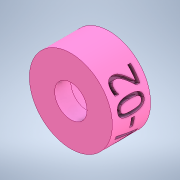
# Autodesk Inventor part: brakeLockSpacer
Saved by Autodesk Inventor 2021.1 (Build 251245000, 245)
## iProperties
Created: 2020-08-18
Part Number: brakeLockSpacer
Material: Polycarbonate, Smoke
Document SubType Name: Modeling
Designer: robst
Density: 1.2 g/cm^3
Appearance: Pink
Author: robst
Autodesk Inventor part; units mm, degrees
ref_plane "XZ Plane" through (0, 0, 0) normal (0, 1, 0) x (-1, 0, 0)
ref_plane "XY Plane" through (0, 0, 0) normal (0, 0, 1) x (1, 0, 0)
sketch "Sketch1" plane through (0, 0, 0) normal (0, 0, 1) x (1, 0, 0)
  circle A0 centre (0, 0) radius 8.0645
  circle A1 centre (0, 0) radius 20.6375
  dimension "d0" = 16.129
  dimension "d1" = 41.275
  constraints: 2 centre point, 2 coincident
  measures "d0" diameter of A0
  measures "d1" diameter of A1
extrude "Extrusion1" add sketch "Sketch1" against normal blind 19.05
sketch "Sketch3" plane through (0, 0, 0) normal (1, 0, 0) x (0, 1, 0)
  line L0 (0, 0) -> (0, -127) construction
  line L1 (-8.0645, -19.05) -> (-8.0645, 0) construction
  line L2 (-20.6375, -19.05) -> (20.6375, -19.05) construction
  line L3 (8.0645, -19.05) -> (8.0645, 0) construction
  line L4 (8.0645, -19.05) -> (8.0645, -8.0515)
  line L5 (8.0645, -8.0515) -> (14.4145, -19.05)
  line L6 (8.0645, -19.05) -> (22.7292, -19.05)
  dimension "d8" = 30
  dimension "d10" = 6.35
  constraints: 8 end point, 1 parallel, 1 point on line, 2 other
  measures "d8" angle of L5 L3
  measures "d10" distance of L5.end L3.start
revolve "Revolution1" cut sketch "Sketch3" angle 360 about axis through (0, 0, 0) along (0, 0, -1)
ref_plane "Work Plane1" through (20.6375, 0, 0) normal (1, 0, 0) x (0, 1, 0)
sketch "Sketch9" plane through (20.6375, 0, 0) normal (1, 0, 0) x (0, 1, 0)
  line L0 (20.6375, 0) -> (20.6375, -19.05) construction
  line L1 (20.6375, -9.525) -> (-20.6375, -9.525) construction
  line L2 (-20.6375, 0) -> (-20.6375, -19.05) construction
  line L3 (-7.4152, -3.175) -> (-11.7892, -15.875)
  line L4 (-11.7892, -15.875) -> (-13.6108, -15.875)
  line L5 (-13.6108, -15.875) -> (-17.9848, -3.175)
  line L6 (-17.9848, -3.175) -> (-16.1735, -3.175)
  line L7 (-16.1735, -3.175) -> (-12.6537, -13.724)
  line L8 (-12.6537, -13.724) -> (-9.1339, -3.175)
  line L9 (-9.1339, -3.175) -> (-7.4152, -3.175)
  line L10 (-1.765, -11.0893) -> (-6.5713, -11.0893)
  line L11 (-6.5713, -11.0893) -> (-6.5713, -9.5456)
  line L12 (-6.5713, -9.5456) -> (-1.765, -9.5456)
  line L13 (-1.765, -9.5456) -> (-1.765, -11.0893)
  spline S0 degree 2 poles (7.8269, -9.525) (7.8269, -12.9419) (5.8406, -16.1426) (3.7719, -16.1426) knots 0 0 0 1 2 2 2
  spline S1 degree 2 poles (3.7719, -16.1426) (1.6724, -16.1426) (-0.2933, -12.8801) (-0.2933, -9.5353) knots 0 0 0 1 2 2 2
  spline S2 degree 2 poles (-0.2933, -9.5353) (-0.2933, -6.0979) (1.693, -2.9177) (3.7719, -2.9177) knots 0 0 0 1 2 2 2
  spline S3 degree 2 poles (3.7719, -2.9177) (5.8611, -2.9177) (7.8269, -6.2111) (7.8269, -9.525) knots 0 0 0 1 2 2 2
  spline S4 degree 2 poles (5.645, -13.3947) (5.892, -12.7669) (6.0979, -10.8321) (6.0979, -9.525) knots 0 0 0 1 2 2 2
  spline S5 degree 2 poles (6.0979, -9.525) (6.0979, -8.2179) (5.892, -6.2934) (5.6347, -5.645) knots 0 0 0 1 2 2 2
  spline S6 degree 2 poles (5.6347, -5.645) (5.3774, -4.9966) (4.4821, -4.3277) (3.7719, -4.3277) knots 0 0 0 1 2 2 2
  spline S7 degree 2 poles (3.7719, -4.3277) (3.0618, -4.3277) (2.1458, -4.9966) (1.8782, -5.6656) knots 0 0 0 1 2 2 2
  spline S8 degree 2 poles (1.8782, -5.6656) (1.6209, -6.314) (1.4357, -8.29) (1.4357, -9.5353) knots 0 0 0 1 2 2 2
  spline S9 degree 2 poles (1.4357, -9.5353) (1.4357, -10.8732) (1.6004, -12.664) (1.868, -13.3638) knots 0 0 0 1 2 2 2
  spline S10 degree 2 poles (1.868, -13.3638) (2.115, -14.0225) (3.0309, -14.7326) (3.7719, -14.7326) knots 0 0 0 1 2 2 2
  spline S11 degree 2 poles (3.7719, -14.7326) (4.4718, -14.7326) (5.3877, -14.0637) (5.645, -13.3947) knots 0 0 0 1 2 2 2
  line L14 (17.285, -15.875) -> (9.453, -15.875)
  line L15 (9.453, -15.875) -> (9.453, -14.0739)
  spline S12 degree 2 poles (9.453, -14.0739) (10.2969, -13.2815) (11.7995, -11.8098) (12.5199, -11.0173) knots 0 0 0 1 2 2 2
  spline S13 degree 2 poles (12.5199, -11.0173) (13.971, -9.4221) (15.0311, -7.5078) (15.0311, -6.4889) knots 0 0 0 1 2 2 2
  spline S14 degree 2 poles (15.0311, -6.4889) (15.0311, -5.9538) (14.7017, -5.151) (14.4033, -4.8937) knots 0 0 0 1 2 2 2
  spline S15 degree 2 poles (14.4033, -4.8937) (14.1048, -4.6364) (13.3226, -4.3791) (12.8492, -4.3791) knots 0 0 0 1 2 2 2
  spline S16 degree 2 poles (12.8492, -4.3791) (12.3964, -4.3791) (11.4701, -4.6056) (11.0482, -4.7805) knots 0 0 0 1 2 2 2
  spline S17 degree 2 poles (11.0482, -4.7805) (10.688, -4.9246) (10.019, -5.3363) (9.8132, -5.4803) knots 0 0 0 1 2 2 2
  line L16 (9.8132, -5.4803) -> (9.7205, -5.4803)
  line L17 (9.7205, -5.4803) -> (9.7205, -3.669)
  spline S18 degree 2 poles (9.7205, -3.669) (10.2454, -3.4117) (12.1288, -2.9074) (12.9727, -2.9074) knots 0 0 0 1 2 2 2
  spline S19 degree 2 poles (12.9727, -2.9074) (14.7532, -2.9074) (16.7601, -4.7908) (16.7601, -6.3963) knots 0 0 0 1 2 2 2
  spline S20 degree 2 poles (16.7601, -6.3963) (16.7601, -7.1476) (16.4102, -8.4032) (16.1014, -8.9384) knots 0 0 0 1 2 2 2
  spline S21 degree 2 poles (16.1014, -8.9384) (15.7927, -9.4941) (14.8973, -10.585) (14.4033, -11.1099) knots 0 0 0 1 2 2 2
  spline S22 degree 2 poles (14.4033, -11.1099) (13.6005, -11.9847) (11.6348, -13.8578) (11.0482, -14.4033) knots 0 0 0 1 2 2 2
  line L18 (11.0482, -14.4033) -> (17.285, -14.4033)
  line L19 (17.285, -14.4033) -> (17.285, -15.875)
  point P0 (0, 0)
  constraints: 2 end point, 2 midpoint, 1 horizontal
emboss "Emboss1" sketch "Sketch9" operation cut depth 2.54 direction (-1, 0, 0) wrap yes faces at (20.3702, -3.3105, -12.7)
equation "\"d0\" = innerDiameter"
equation "\"d1\" = outsideDiameter"
equation "\"d8\" = brakeHandle"
equation "\"d10\" = heightOfBrake"
equation "\"handleDiameter\" = 101.6"
equation "\"brakeHandle\" = 30deg"
equation "\"innerDiameter\" = 16.129"
equation "\"heightOfBrake\" = 6.35"
equation "\"outsideDiameter\" = 41.275"
equation "\"d36\" = 0.5 * outsideDiameter"
body "Solid1"
